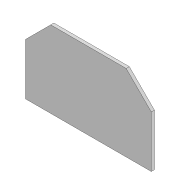
# Autodesk Inventor part: PSM_ECover
Saved by Autodesk Inventor 2022 (Build 260153000, 153)
## iProperties
Created: 2022-12-21
Part Number: PSM_ECover
Material: Generisch
Document SubType Name: Modeling
Designer: alexw
Density: 1 g/cm^3
Appearance: Vorgabe
Author: alexw
Autodesk Inventor part; units mm, degrees
ref_plane "YZ Plane" through (0, 0, 0) normal (1, 0, 0) x (0, 1, 0)
ref_plane "XZ Plane" through (0, 0, 0) normal (0, 1, 0) x (-1, 0, 0)
ref_plane "XY Plane" through (0, 0, 0) normal (0, 0, 1) x (1, 0, 0)
sketch "Skizze1" plane through (0, 0, 0) normal (0, 0, 1) x (1, 0, 0)
  line L0 (-100, 61) -> (100, 61)
  line L1 (100, 61) -> (100, -61)
  line L2 (100, -61) -> (-100, -61)
  line L3 (-100, -61) -> (-100, 61)
  line L4 (-100, 61) -> (100, -61) construction
  line L5 (100, 61) -> (-100, -61) construction
  line L6 (-100, 21) -> (-60, 61)
  line L7 (60, 61) -> (100, 21)
  point P0 (0, 0)
  dimension "d0" = 45
  dimension "d1" = 40
  dimension "d2" = 122
  dimension "d3" = 200
  dimension "d4" = 40
  dimension "d5" = 45
  constraints: 16 end point, 4 point on line, 2 midpoint, 2 parallel, 1 horizontal, 1 perpendicular
  measures "d0" angle of L3 L6
  measures "d1" distance from line of L6.end L3
  measures "d2" distance of L2.end L0.start
  measures "d3" distance of L1.end L2.end
  measures "d4" distance of L0.end L7.start
  measures "d5" angle of L1 L7
extrude "Extrusion1" add sketch "Skizze1" along normal blind 5 contours L0 L7 L1 L2 L3 L6
